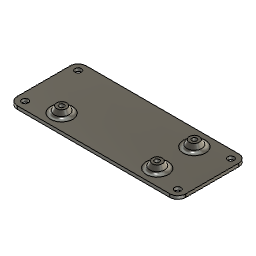
pcb sled (Autodesk Fusion 360 design; units mm, degrees)
Autodesk Fusion 360 part; units mm, degrees
sketch "Sketch1" plane through (0, 0, 0) normal (0, 0, 1) x (1, 0, 0)
  line L0 (36.5125, -12.7) -> (-36.5125, -12.7) construction
  line L1 (-36.5125, -12.7) -> (-36.5125, 12.7) construction
  line L2 (-36.5125, 12.7) -> (36.5125, 12.7) construction
  line L3 (36.5125, 12.7) -> (36.5125, -12.7) construction
  line L4 (36.5125, -12.7) -> (-36.5125, 12.7) construction
  line L5 (-36.5125, -12.7) -> (36.5125, 12.7) construction
  line L6 (40.3225, -16.51) -> (-40.3225, -16.51)
  line L7 (-40.3225, -16.51) -> (-40.3225, 16.51)
  line L8 (-40.3225, 16.51) -> (40.3225, 16.51)
  line L9 (40.3225, 16.51) -> (40.3225, -16.51)
  circle A0 centre (-36.5125, 12.7) radius 1.524
  circle A1 centre (36.5125, 12.7) radius 1.524
  circle A2 centre (-36.5125, -12.7) radius 1.524
  circle A3 centre (36.5125, -12.7) radius 1.524
  line L10 (22.86, -8.89) -> (-22.86, -8.89) construction
  line L11 (-22.86, -8.89) -> (-22.86, 8.89) construction
  line L12 (-22.86, 8.89) -> (22.86, 8.89) construction
  line L13 (22.86, 8.89) -> (22.86, -8.89) construction
  line L14 (22.86, -8.89) -> (-22.86, 8.89) construction
  line L15 (-22.86, -8.89) -> (22.86, 8.89) construction
  circle A4 centre (-22.86, 8.89) radius 1.143
  circle A5 centre (22.86, 8.89) radius 1.143
  circle A6 centre (-22.86, -8.89) radius 1.143
  circle A7 centre (22.86, -8.89) radius 1.143
  circle A8 centre (-22.86, 8.89) radius 2.413
  circle A9 centre (22.86, 8.89) radius 2.413
  circle A10 centre (-22.86, -8.89) radius 2.413
  circle A11 centre (22.86, -8.89) radius 2.413
  dimension "d1" = 73.025
  dimension "d2" = 25.4
  dimension "d3" = -3.81
  dimension "d4" = 3.048
  dimension "d7" = 73.025
  dimension "d8" = -25.4
  dimension "d9" = 45.72
  dimension "d10" = 17.78
  dimension "d11" = 2.286
  dimension "d14" = 45.72
  dimension "d15" = -17.78
  dimension "d16" = 1.27
  dimension "d17" = 1.27
  dimension "d18" = 1.27
  dimension "d19" = 1.27
  constraint horizontal L0
  constraint perpendicular L0 L1
  constraint parallel L0 L2
  constraint parallel L1 L3
  constraint coincident L4 origin
  constraint coincident L5 origin
  constraint coincident L1.end L2.start
  constraint horizontal L10
  constraint perpendicular L10 L11
  constraint parallel L10 L12
  constraint parallel L11 L13
  constraint coincident L14 origin
  constraint coincident L15 origin
  constraint coincident L11.end L12.start
  measures "d1" distance of L1.end L2.end
  measures "d2" distance of L0.end L1.end
  measures "d4" diameter of A0
  measures "d9" distance of L11.end L12.end
  measures "d10" distance of L10.end L11.end
  measures "d11" diameter of A4
extrude "Extrude1" add sketch "Sketch1" along normal blind 1.5 contours L6 L7 L8 L9 | A4 | A8 | A9 | A10 | A11
extrude "Extrude2" add sketch "Sketch1" along normal blind 4.5 contours A9 | A10 | A11
draft "Draft1" angle 30 neutral plane through (0, 0, 4.5) pull (0, 0, 1) 3 faces at (-20.459, -8.6497, 2.5) (25.261, 9.1303, 2.5) (25.261, -8.6497, 2.5)
fillet "Fillet1" radius 3.81 4 edges at (-40.3225, -16.51, 0.75) (-40.3225, 16.51, 0.75) (40.3225, 16.51, 0.75) (40.3225, -16.51, 0.75)
fillet "Fillet2" radius 2 3 edges at (-26.7245, -7.3911, 1.5) (18.9955, -7.3911, 1.5) (18.9955, 10.3889, 1.5)
